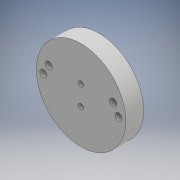
# Autodesk Inventor part: cABEZOTE
Saved by Autodesk Inventor 2017 (Build 210142000, 142)
## iProperties
Created: 2021-07-26
Part Number: cABEZOTE
Material: Generic
Document SubType Name: Modeling
Designer: USUARIO
Density: 1 g/cm^3
Appearance: Default
Author: USUARIO
Autodesk Inventor part; units mm, degrees
ref_plane "YZ Plane" through (0, 0, 0) normal (1, 0, 0) x (0, 1, 0)
ref_plane "XZ Plane" through (0, 0, 0) normal (0, 1, 0) x (-1, 0, 0)
ref_plane "XY Plane" through (0, 0, 0) normal (0, 0, 1) x (1, 0, 0)
sketch "Sketch1" plane through (0, 0, 0) normal (0, 1, 0) x (-1, 0, 0)
  circle A0 centre (0, 0) radius 25
  dimension "d0" = 50
  constraints: 1 centre point, 1 coincident
  measures "d0" diameter of A0
extrude "Extrusion1" add sketch "Sketch1" along normal blind 10
sketch "Sketch2" plane through (0, 10, 0) normal (0, 1, 0) x (1, 0, 0)
  circle A0 centre (0, -5.5) radius 1.5
  circle A1 centre (0, 5.5) radius 1.5
  circle A2 centre (-18, -5.5) radius 2
  circle A3 centre (-21, 0) radius 2
  circle A4 centre (21, 0) radius 2
  circle A5 centre (18, -5.5) radius 2
  point P0 (0, 0)
  dimension "d3" = 3
  dimension "d4" = 3
  dimension "d5" = 5.5
  dimension "d6" = 5.5
  dimension "d7" = 4
  dimension "d8" = 4
  dimension "d9" = 4
  dimension "d10" = 4
  dimension "d11" = 21
  dimension "d12" = 21
  dimension "d13" = 18
  dimension "d14" = 18
  constraints: 6 centre point
  measures "d3" diameter of A0
  measures "d4" diameter of A1
  measures "d5" distance of point (0, 0) A0.centre
  measures "d6" distance of point (0, 0) A1.centre
  measures "d7" diameter of A2
  measures "d8" diameter of A3
  measures "d9" diameter of A4
  measures "d10" diameter of A5
  measures "d11" distance of A4.centre point (0, 0)
  measures "d12" distance of point (0, 0) A3.centre
  measures "d13" distance of A0.centre A2.centre
  measures "d14" distance of A0.centre A5.centre
extrude "Extrusion2" cut sketch "Sketch2" against normal blind 10
body "Solid1"
